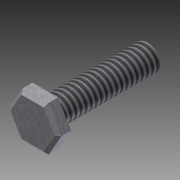
# Autodesk Inventor part: 1_bolt_.25_20
Saved by Autodesk Inventor 2011 (Build 150239000, 239)
## iProperties
Created: 2013-01-17
Part Number: 1_bolt_.25_20
Document SubType Name: Modeling
Designer: Christopher
Density: 1 g/cm^3
Author: Christopher
Autodesk Inventor part; units mm, degrees
ref_plane "YZ Plane" through (0, 0, 0) normal (1, 0, 0) x (0, 1, 0)
ref_plane "XZ Plane" through (0, 0, 0) normal (0, 1, 0) x (-1, 0, 0)
ref_plane "XY Plane" through (0, 0, 0) normal (0, 0, 1) x (1, 0, 0)
sketch "Sketch1" plane through (0, 0, 0) normal (0, 0, 1) x (1, 0, 0)
  circle A0 centre (0, 0) radius 3.175
  line L0 (3.2079, 5.5563) -> (6.4158, 0)
  line L1 (6.4158, 0) -> (3.2079, -5.5562)
  line L2 (3.2079, -5.5562) -> (-3.2079, -5.5562)
  line L3 (-3.2079, -5.5562) -> (-6.4158, 0)
  line L4 (-6.4158, 0) -> (-3.2079, 5.5563)
  line L5 (-3.2079, 5.5563) -> (3.2079, 5.5563)
  dimension "d0" = 6.35
  dimension "d1" = 11.1125
  constraints: 12 end point, 2 coincident, 1 centre point, 1 horizontal, 13 other
  measures "d0" diameter of A0
  measures "d1" distance between parallel lines of L5 L2
extrude "Extrusion1" add sketch "Sketch1" against normal blind 25.4 contours A0
extrude "Extrusion2" add sketch "Sketch1" along normal blind 3.175 contours A0 | L0 L1 L2 L3 L4 L5
thread "Thread1" size "1/4-20 UNC" class "2A" standard "ANSI Unified Screw Threads" full length
chamfer "Chamfer1" distance 0.7937 angle 45 6 edges at (4.8119, 2.7781, 3.175) (0, 5.5563, 3.175) (-4.8119, 2.7781, 3.175) (-4.8119, -2.7781, 3.175) (0, -5.5562, 3.175) (4.8119, -2.7781, 3.175)
body "Solid1"
